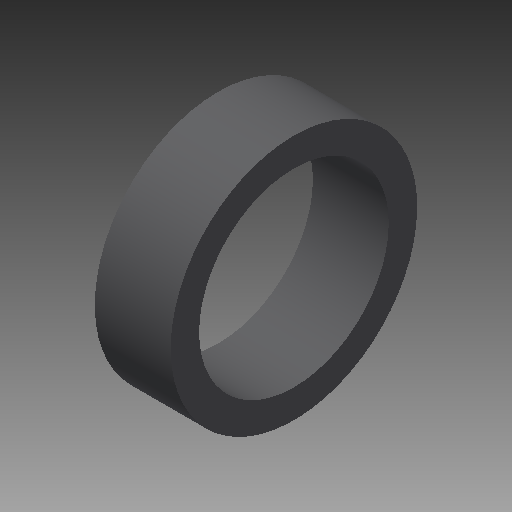
# Autodesk Inventor part: BK 15collar
Saved by Autodesk Inventor 2018 (Build 220112000, 112)
## iProperties
Category: PARTsolutions
Company: THK
Created: 2017-05-30
Part Number: BK 15collar
Catalog Web Link: www.cadenas.de
Description: Collar BK-
Vendor: THK
Document SubType Name: Modeling
Designer: psAdmin
Manufacturer: THK
Mass: 0.731598 g
Surface Area: 8.94176 cm^2
Volume: 0.731598 cm^3
Density: 1 g/cm^3
Material: Generic
Appearance: PSOLRGB-192-192-192
PSOL_IDENT_0: {$CADENAS_DATA\23d-libs\thk\fed_screw\ball_screw\ball_screw_peripheral\suport_unit\fixed_side_type_b
PSOL_IDENT_1: k_collar.prj},167 {VTYP=3D},{NB=BK 15collar},{LINA=BK 15collar},{NN=Collar BK},{DATE=16.05.2017 06:0
PSOL_IDENT_2: 9:49},{GEOMDATE=12.10.2012 10:34:00},{VERSION=},{LINEID=30},{LINESUBID=-1},{WBVAR=}  {NB=BK 15collar
PSOL_IDENT_3: },{LINA=BK 15collar},{KT=DUMMY},{MN=BK 15},{DO=19.5},{DI=15},{T=6.0}
NN: Collar BK
NB: BK 15collar
NBSYN: $MN.collar
LINA: BK 15collar
MN: BK 15
DO: 19.5
DI: 15
T: 6.0
SUPPLIER: THK
ARTICLENO: BK 15collar
BOMINFO: BK 15collar
CREATOR: CADENAS GmbH
Title: BK 15collar
Author: Cadenas PARTsolutions
Autodesk Inventor part; units mm, degrees
ref_plane "YZ Plane" through (0, 0, 0) normal (1, 0, 0) x (0, 1, 0)
ref_plane "XZ Plane" through (0, 0, 0) normal (0, 1, 0) x (-1, 0, 0)
ref_plane "XY Plane" through (0, 0, 0) normal (0, 0, 1) x (1, 0, 0)
sketch "Sketch_1" plane through (0, 0, 0) normal (0, 0, 1) x (1, 0, 0)
  line L0 (6, 0) -> (0, 0)
  line L1 (0, 7.5) -> (6, 7.5)
  line L2 (6, 7.5) -> (6, 9.75)
  line L3 (6, 9.75) -> (0, 9.75)
  line L4 (0, 9.75) -> (0, 7.5)
  constraints: 10 end point
revolve "Revolution1" add sketch "Sketch_1" angle 360 about axis through (6, 0, 0) along (1, 0, 0)
ref_plane "collar_XY" through (0, 0, 0) normal (1, 0, 0) x (0, 0, -1)
ref_plane "collar_YZ" through (0, 0, 0) normal (0, 0, -1) x (0, 1, 0)
ref_plane "collar_ZX" through (0, 0, 0) normal (0, 1, 0) x (1, 0, 0)
body "Solid1"
